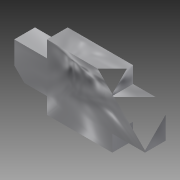
# Autodesk Inventor part: ColdFingerStem
Saved by Autodesk Inventor 2014 (Build 180170000, 170)
## iProperties
Created: 2015-04-18
Part Number: ColdFingerStem
Material: Generic
Document SubType Name: Modeling
Designer: Owner
Density: 1 g/cm^3
Appearance: Aluminum - Polished
Author: Owner
Autodesk Inventor part; units mm, degrees
ref_plane "YZ Plane" through (0, 0, 0) normal (1, 0, 0) x (0, 1, 0)
ref_plane "XZ Plane" through (0, 0, 0) normal (0, 1, 0) x (-1, 0, 0)
ref_plane "XY Plane" through (0, 0, 0) normal (0, 0, 1) x (1, 0, 0)
sketch "Sketch1" plane through (0, 0, 0) normal (0, 0, 1) x (1, 0, 0)
  line L0 (-3.3239, 4.8371) -> (16.6761, 4.8371)
  line L1 (16.6761, 4.8371) -> (16.6761, -15.1629)
  line L2 (16.6761, -15.1629) -> (-3.3239, -15.1629)
  line L3 (-3.3239, -15.1629) -> (-3.3239, 4.8371)
  line L4 (14.5634, -0.1629) -> (29.6761, -0.1629)
  line L5 (29.6761, -0.1629) -> (29.6761, -10.1629)
  line L6 (29.6761, -10.1629) -> (14.5634, -10.1629)
  line L7 (14.5634, -10.1629) -> (14.5634, -0.1629)
  line L8 (-1.0107, -0.1629) -> (-16.3239, -0.1629)
  line L9 (-16.3239, -0.1629) -> (-16.3239, -10.1629)
  line L10 (-16.3239, -10.1629) -> (-1.0107, -10.1629)
  line L11 (-1.0107, -10.1629) -> (-1.0107, -0.1629)
  line L12 (-3.3239, 4.8371) -> (-8.3239, -0.1629)
  line L13 (16.6761, 4.8371) -> (21.6761, -0.1629)
  line L14 (-3.3239, -15.1629) -> (-8.3239, -10.1629)
  line L15 (16.6761, -15.1629) -> (21.6761, -10.1629)
  point P0 (0, 0)
  dimension "d0" = 20
  dimension "d1" = 20
  dimension "d2" = 10
  dimension "d3" = 10
  dimension "d4" = 0
  dimension "d5" = 5
  dimension "d6" = 13
  dimension "d7" = 13
  dimension "d10" = 45
  dimension "d11" = 45
  dimension "d12" = 45
  constraints: 32 end point, 7 parallel, 4 point on line, 3 horizontal, 3 perpendicular
  measures "d0" distance of L0.start L0.end
  measures "d1" distance of L0.end L1.end
  measures "d2" distance of L4.end L5.end
  measures "d3" distance of L8.end L9.end
  measures "d4" distance between parallel lines of L8 L4
  measures "d5" distance between parallel lines of L2 L6
  measures "d6" distance between parallel lines of L3 L9
  measures "d7" distance between parallel lines of L1 L5
  measures "d10" angle of L3 L12
  measures "d11" angle of L3 L14
  measures "d12" angle of L15 L1
extrude "Extrusion1" add sketch "Sketch1" along normal blind 6.35
body "Solid1"
